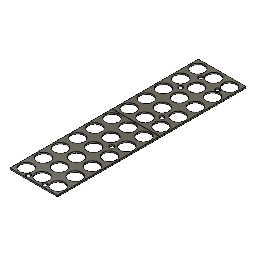
11x3_pcb_mask (Autodesk Fusion 360 design; units mm, degrees)
Autodesk Fusion 360 part; units mm, degrees
sketch "11x3-Edge_Cuts" plane through (0, 0, 0) normal (0, 0, 1) x (1, 0, 0)
  line L0 (48.54, -24.51) -> (48.54, -285.21)
  line L1 (114.54, -24.51) -> (48.54, -24.51)
  line L2 (114.54, -285.21) -> (114.54, -24.51)
  line L3 (48.54, -285.21) -> (114.54, -285.21)
sketch "11x3-User_Drawings" plane through (0, 0, 0) normal (0, 0, 1) x (1, 0, 0)
  circle A0 centre (81.6168, -131.26) radius 9
  circle A1 centre (81.6168, -107.56) radius 9
  circle A2 centre (59.6168, -226.06) radius 9
  circle A3 centre (81.6168, -178.66) radius 9
  circle A4 centre (81.6168, -202.36) radius 9
  circle A5 centre (59.6168, -178.66) radius 9
  circle A6 centre (59.6168, -131.26) radius 9
  circle A7 centre (103.617, -83.86) radius 9
  circle A8 centre (103.617, -60.16) radius 9
  circle A9 centre (103.617, -154.96) radius 9
  circle A10 centre (81.6168, -83.86) radius 9
  circle A11 centre (59.6168, -273.46) radius 9
  circle A12 centre (103.617, -36.46) radius 9
  circle A13 centre (103.617, -226.06) radius 9
  circle A14 centre (81.6168, -60.16) radius 9
  circle A15 centre (103.617, -131.26) radius 9
  circle A16 centre (81.6168, -226.06) radius 9
  circle A17 centre (103.617, -107.56) radius 9
  circle A18 centre (59.6168, -202.36) radius 9
  circle A19 centre (68.58, -272.288) radius 0.000001
  circle A20 centre (81.6168, -154.96) radius 9
  circle A21 centre (81.6168, -249.76) radius 9
  circle A22 centre (59.6168, -249.76) radius 9
  circle A23 centre (81.6168, -273.46) radius 9
  circle A24 centre (103.617, -202.36) radius 9
  circle A25 centre (59.6168, -60.16) radius 9
  circle A26 centre (59.6168, -36.46) radius 9
  circle A27 centre (103.617, -273.46) radius 9
  circle A28 centre (81.6168, -36.46) radius 9
  circle A29 centre (59.6168, -107.56) radius 9
  circle A30 centre (59.6168, -83.86) radius 9
  circle A31 centre (103.617, -249.76) radius 9
  circle A32 centre (59.6168, -154.96) radius 9
  circle A33 centre (103.617, -178.66) radius 9
sketch "11x3-User_Comments" plane through (0, 0, 0) normal (0, 0, 1) x (1, 0, 0)
  circle A0 centre (93.472, -188.976) radius 3
  circle A1 centre (93.16, -119.63) radius 3
  circle A2 centre (92.63, -280.65) radius 3
  circle A3 centre (98.9, -48.06) radius 3
  circle A4 centre (72.39, -45.212) radius 3
  circle A5 centre (70.104, -70.612) radius 3
  circle A6 centre (70.104, -280.924) radius 3
extrude "Extrude1" add sketch "11x3-Edge_Cuts" along normal blind 2 contours L0 L1 L2 L3 picked at (92.54, -198.31) makes body 1
extrude "Extrude2" cut sketch "11x3-User_Drawings" sketch "11x3-User_Comments" along normal blind 2 contours A0 | A1 | A2 | A3 | A4 | A5 | A6 | A7 | A8 | A9 | A10 | A11 | A12 | A13 | A14 | A15 | A16 | A17 | A18 | A20 | A21 | A22 | A23 | A24 | A25 | A26 | A27 | A28 | A29 | A30 | A31 | A32 | A33 picked at (84.768087, -132.561651) picked at (77.693454, -105.125947) picked at (62.095516, -224.37004) picked at (84.768087, -179.961651) picked at (84.768087, -203.661651) picked at (62.095516, -176.97004) picked at (60.712823, -128.467379) picked at (99.414093, -81.776505) picked at (102.117, -57.561924) picked at (106.768287, -156.261651) picked at (77.693454, -81.425947) picked at (58.520777, -276.252621) picked at (102.077604, -33.600551) picked at (106.768287, -227.361651) picked at (80.1168, -57.561924) picked at (106.768287, -132.561651) picked at (84.768087, -227.361651) picked at (99.414093, -105.476505) picked at (62.095516, -200.67004) picked at (84.768087, -156.261651) picked at (81.84099, -252.617956) picked at (62.707709, -247.652654) picked at (80.949237, -270.535216) picked at (106.768287, -203.661651) picked at (61.387495, -59.145898) picked at (61.875271, -33.308811) picked at (102.949437, -270.535216) picked at (80.077404, -33.600551) picked at (58.150308, -105.409051) picked at (58.150308, -81.709051) picked at (103.84119, -252.617956) picked at (62.095516, -153.27004) picked at (106.768287, -179.961651) of sketch 2 contours A0 | A1 | A2 | A3 | A4 | A5 | A6 picked at (94.416404, -188.830287) picked at (93.239701, -120.560874) picked at (91.63, -279.52336) picked at (99.720914, -47.094986) picked at (73.210914, -44.246986) picked at (71.504615, -70.906755) picked at (69.104, -279.79736) bodies 1
move_body "Move1" bodies 1 to x (1, 0, 0) y (0, 1, 0) z (0, 0, 1) at (0, 144, 0)
split "Split1" by plane through (0, 0, 0) normal (0, 1, 0) bodies 1 makes body 2 at (91.149356, 73.899482, 0)
